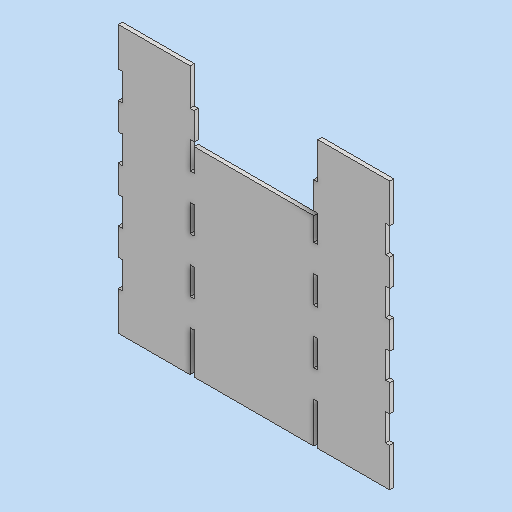
# Autodesk Inventor part: back plate
Saved by Autodesk Inventor 2026 (Build 300175000, 175)
## iProperties
Created: 2026-02-11
Part Number: back plate
Material: Generic
Document SubType Name: Modeling
Designer: mones
Density: 1 g/cm^3
Appearance: Default
Author: mones
Autodesk Inventor part; units mm, degrees
ref_plane "YZ Plane" through (0, 0, 0) normal (1, 0, 0) x (0, 1, 0)
ref_plane "XZ Plane" through (0, 0, 0) normal (0, 1, 0) x (-1, 0, 0)
ref_plane "XY Plane" through (0, 0, 0) normal (0, 0, 1) x (1, 0, 0)
sketch "Sketch1" plane through (0, 0, 0) normal (0, 0, 1) x (1, 0, 0)
  line L0 (-100, 98.5) -> (100, -98.5) construction
  line L1 (100, 98.5) -> (-100, -98.5) construction
  line L2 (-100, 98.5) -> (-100, 70)
  line L3 (-100, 50) -> (-100, 30)
  line L4 (-100, 10) -> (-100, -10)
  line L5 (-100, -30) -> (-100, -50)
  line L6 (-100, -70) -> (-100, -98.5)
  line L7 (-100, 98.5) -> (-100, 95.5)
  line L8 (-100, 98.5) -> (-100, 95.5)
  line L9 (-100, 98.5) -> (-97, 98.5)
  line L10 (-100, -70) -> (-97, -70)
  line L11 (-100, -50) -> (-97, -50)
  line L12 (-100, -30) -> (-97, -30)
  line L13 (-100, -10) -> (-97, -10)
  line L14 (-100, 10) -> (-97, 10)
  line L15 (-100, 30) -> (-97, 30)
  line L16 (-100, 50) -> (-97, 50)
  line L17 (-100, 70) -> (-97, 70)
  line L18 (-100, -98.5) -> (-100, -70)
  line L19 (-100, -50) -> (-100, -30)
  line L20 (-100, -10) -> (-100, 10)
  line L21 (-100, 30) -> (-100, 50)
  line L22 (-100, 70) -> (-100, 98.5)
  line L23 (100, 98.5) -> (97, 98.5)
  line L24 (100, -98.5) -> (100, -70)
  line L25 (100, -50) -> (100, -30)
  line L26 (100, -10) -> (100, 10)
  line L27 (100, 30) -> (100, 50)
  line L28 (100, 70) -> (97, 70)
  line L29 (100, 50) -> (97, 50)
  line L30 (100, 30) -> (97, 30)
  line L31 (100, 10) -> (97, 10)
  line L32 (100, -10) -> (97, -10)
  line L33 (100, -30) -> (97, -30)
  line L34 (100, -50) -> (97, -50)
  line L35 (100, -70) -> (97, -70)
  line L36 (100, -70) -> (100, -98.5)
  line L37 (100, -30) -> (100, -50)
  line L38 (100, 10) -> (100, -10)
  line L39 (100, 98.5) -> (100, 70)
  line L40 (100, 50) -> (100, 30)
  line L41 (-97, -98.5) -> (-47, -98.5)
  line L42 (-47, -98.5) -> (-47, -68.5)
  line L43 (-47, -48.5) -> (-47, -28.5)
  line L44 (-47, -8.5) -> (-47, 11.5)
  line L45 (-47, 31.5) -> (-47, 51.5)
  line L46 (-47, 71.5) -> (-47, 98.5)
  line L47 (-47, 71.5) -> (-44, 71.5)
  line L48 (-47, 51.5) -> (-44, 51.5)
  line L49 (-47, 31.5) -> (-44, 31.5)
  line L50 (-47, 11.5) -> (-44, 11.5)
  line L51 (-47, -8.5) -> (-44, -8.5)
  line L52 (-47, -28.5) -> (-44, -28.5)
  line L53 (-47, -68.5) -> (-44, -68.5)
  line L54 (-47, -98.5) -> (-100, -98.5)
  line L55 (-44, -28.5) -> (-44, -48.5)
  line L56 (-44, -48.5) -> (-47, -48.5)
  line L57 (-44, -98.5) -> (-44, -68.5)
  line L58 (-47, -68.5) -> (-47, -98.5)
  line L59 (-44, -48.5) -> (-44, -28.5)
  line L60 (-47, -28.5) -> (-47, -48.5)
  line L61 (-44, -8.5) -> (-44, 11.5)
  line L62 (-47, 11.5) -> (-47, -8.5)
  line L63 (-44, 31.5) -> (-44, 48.5)
  line L64 (-47, 98.5) -> (-47, 71.5)
  line L65 (-47, 51.5) -> (-47, 31.5)
  line L66 (-100, 98.5) -> (-47, 98.5)
  line L67 (100, -98.5) -> (47, -98.5)
  line L68 (47, -98.5) -> (47, -68.5)
  line L69 (47, -48.5) -> (47, -28.5)
  line L70 (47, -8.5) -> (47, 11.5)
  line L71 (47, 31.5) -> (47, 51.5)
  line L72 (47, 71.5) -> (47, 98.5)
  line L73 (47, 71.5) -> (44, 71.5)
  line L74 (47, 51.5) -> (44, 51.5)
  line L75 (47, 31.5) -> (44, 31.5)
  line L76 (47, 11.5) -> (44, 11.5)
  line L77 (47, -8.5) -> (44, -8.5)
  line L78 (47, -28.5) -> (44, -28.5)
  line L79 (47, -68.5) -> (44, -68.5)
  line L80 (44, -28.5) -> (44, -48.5)
  line L81 (44, -48.5) -> (47, -48.5)
  line L82 (44, -98.5) -> (44, -68.5)
  line L83 (47, -68.5) -> (47, -98.5)
  line L84 (44, -48.5) -> (44, -28.5)
  line L85 (47, -28.5) -> (47, -48.5)
  line L86 (44, -8.5) -> (44, 11.5)
  line L87 (47, 11.5) -> (47, -8.5)
  line L88 (44, 31.5) -> (44, 48.5)
  line L89 (47, 98.5) -> (47, 71.5)
  line L90 (47, 51.5) -> (47, 31.5)
  line L91 (100, -98.5) -> (47, -98.5)
  line L92 (44, -98.5) -> (-44, -98.5)
  line L93 (47, 98.5) -> (97, 98.5)
  line L94 (47, 98.5) -> (100, 98.5)
  line L95 (-97, 98.5) -> (-47, 98.5)
  line L96 (-97, 70) -> (-97, 50)
  line L97 (-97, 30) -> (-97, 10)
  line L98 (-97, -10) -> (-97, -30)
  line L99 (-97, -50) -> (-97, -70)
  line L100 (97, -50) -> (97, -70)
  line L101 (97, -10) -> (97, -30)
  line L102 (97, 30) -> (97, 10)
  line L103 (97, 70) -> (97, 50)
  line L104 (44, 71.5) -> (44, 51.5)
  line L105 (44, 48.5) -> (-44, 48.5)
  line L106 (-44, 71.5) -> (-44, 51.5)
  point P0 (0, 0)
  constraints: 214 end point, 100 perpendicular, 37 parallel, 7 collinear, 4 point on line, 3 horizontal, 2 midpoint
extrude "Extrusion1" add sketch "Sketch1" along normal blind 3
body "Solid1"
